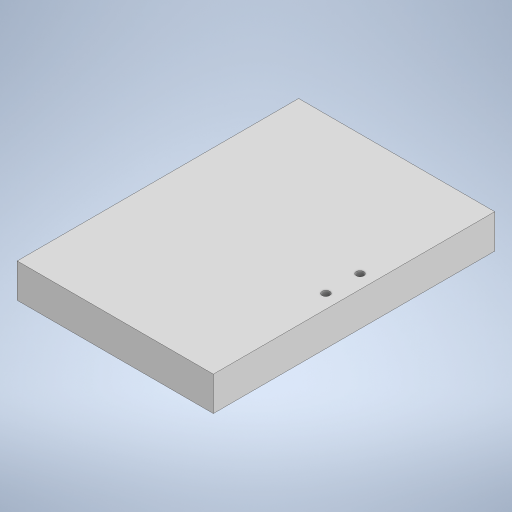
# Autodesk Inventor part: PCB
Saved by Autodesk Inventor 2024.2 (Build 282272000, 272)
## iProperties
Created: 2024-02-18
Part Number: PCB
Material: Generic
Document SubType Name: Modeling
Designer: kdcao
Density: 1 g/cm^3
Appearance: Default
Author: kdcao
Autodesk Inventor part; units mm, degrees
ref_plane "YZ Plane" through (0, 0, 0) normal (1, 0, 0) x (0, 1, 0)
ref_plane "XZ Plane" through (0, 0, 0) normal (0, 1, 0) x (-1, 0, 0)
ref_plane "XY Plane" through (0, 0, 0) normal (0, 0, 1) x (1, 0, 0)
sketch "Sketch1" plane through (0, 0, 0) normal (0, 1, 0) x (-1, 0, 0)
  line L0 (-28.75, 41.25) -> (28.75, 41.25)
  line L1 (28.75, 41.25) -> (28.75, -41.25)
  line L2 (28.75, -41.25) -> (-28.75, -41.25)
  line L3 (-28.75, -41.25) -> (-28.75, 41.25)
  line L4 (-28.75, 41.25) -> (28.75, -41.25) construction
  line L5 (28.75, 41.25) -> (-28.75, -41.25) construction
  point P0 (0, 0)
  dimension "d1" = 82.5
  dimension "d2" = 57.5
  constraints: 12 end point, 2 midpoint, 2 parallel, 1 horizontal, 1 perpendicular
  measures "d1" distance of L0.end L1.end
  measures "d2" distance of L0.start L0.end
extrude "Extrusion1" add sketch "Sketch1" along normal blind 10
sketch "Sketch2" plane through (0, 10, 0) normal (0, 1, 0) x (1, 0, 0)
  line L0 (-28.75, -41.25) -> (28.75, -41.25) projected
  line L1 (28.75, -41.25) -> (28.75, 41.25) projected
  point P0 (0, 0)
  point P1 (24.75, -4.25)
  point P2 (24.75, 5.75)
  dimension "d12" = 37
  dimension "d13" = 10
  dimension "d14" = 4
  dimension "d15" = 4
  measures "d12" distance from line of L0 point (24.75, -4.25)
  measures "d13" distance of point (24.75, 5.75) point (24.75, -4.25)
  measures "d14" distance from line of L1 point (24.75, -4.25)
  measures "d15" distance from line of L1 point (24.75, 5.75)
hole "Hole1" at (24.75, 10, -5.75) at (24.75, 10, 4.25) direction (0, -1, 0) diameter 2.2 end through all
body "Solid1"
